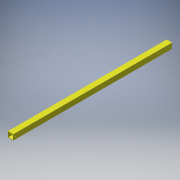
# Autodesk Inventor part: Long Side
Saved by Autodesk Inventor 2017 (Build 210142000, 142)
## iProperties
Created: 2017-01-16
Part Number: Long Side
Material: Generic
Document SubType Name: Modeling
Designer: Ben
Density: 1 g/cm^3
Appearance: Smooth - Yellow
Author: Ben
Autodesk Inventor part; units mm, degrees
ref_plane "YZ Plane" through (0, 0, 0) normal (1, 0, 0) x (0, 1, 0)
ref_plane "XZ Plane" through (0, 0, 0) normal (0, 1, 0) x (-1, 0, 0)
ref_plane "XY Plane" through (0, 0, 0) normal (0, 0, 1) x (1, 0, 0)
sketch "Sketch1" plane through (0, 0, 0) normal (0, 0, 1) x (1, 0, 0)
  line L0 (0, 0) -> (-11.1125, 0) construction
  line L1 (0, 0) -> (0, 11.1125) construction
  line L2 (-11.1125, 11.1125) -> (11.1125, 11.1125)
  line L3 (11.1125, 11.1125) -> (11.1125, -11.1125)
  line L4 (11.1125, -11.1125) -> (-11.1125, -11.1125)
  line L5 (-11.1125, -11.1125) -> (-11.1125, 11.1125)
  line L6 (-12.7, 12.7) -> (12.7, 12.7)
  line L7 (12.7, 12.7) -> (12.7, -12.7)
  line L8 (12.7, -12.7) -> (-12.7, -12.7)
  line L9 (-12.7, -12.7) -> (-12.7, 12.7)
  line L10 (-11.1125, 0) -> (-12.7, 0) construction
  line L11 (0, 11.1125) -> (0, 12.7) construction
  dimension "d0" = 25.4
  dimension "d1" = 1.5875
  constraints: 24 end point, 4 horizontal, 4 midpoint, 4 parallel, 4 perpendicular, 2 vertical
  measures "d0" distance of L8.end L6.start
  measures "d1" distance of L1.end L11.end
extrude "Extrusion1" add sketch "Sketch1" along normal mid plane 749.3
sketch "Sketch2" plane through (12.7, -12.7, 374.65) normal (1, 0, 0) x (0, 0, -1)
  line L0 (374.65, 12.7) -> (374.65, 0) construction
  line L1 (0, 0) -> (749.3, 0) construction
  line L2 (0, 12.7) -> (374.65, 12.7) construction
  circle A0 centre (9.525, 12.7) radius 1.27
  circle A1 centre (28.575, 12.7) radius 1.27
  circle A2 centre (739.775, 12.7) radius 1.27
  circle A3 centre (720.725, 12.7) radius 1.27
  dimension "d4" = 2.54
  dimension "d5" = 19.05
  dimension "d6" = 9.525
  constraints: 4 centre point, 4 end point, 2 point on line, 2 symmetric about line, 1 equal radius, 1 midpoint, 1 perpendicular, 2 other
  measures "d4" diameter of A0
  measures "d5" distance of A0.centre A1.centre
  measures "d6" horizontal distance of L1.start A0.centre
extrude "Extrusion2" cut sketch "Sketch2" against normal through all
body "Solid1"
